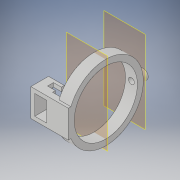
# Autodesk Inventor part: Dc_Ring
Saved by Autodesk Inventor 2019 (Build 230136000, 136)
## iProperties
Created: 2019-10-14
Part Number: Dc_Ring
Material: Generic
Document SubType Name: Modeling
Designer: James
Density: 1 g/cm^3
Appearance: Default
Author: James
Autodesk Inventor part; units mm, degrees
ref_plane "YZ Plane" through (0, 0, 0) normal (1, 0, 0) x (0, 1, 0)
ref_plane "XZ Plane" through (0, 0, 0) normal (0, 1, 0) x (-1, 0, 0)
sketch "Sketch1" plane through (0, 0, 0) normal (1, 0, 0) x (0, 1, 0)
  circle A0 centre (0, 0) radius 16
  circle A1 centre (0, 0) radius 19
  point P0 (19, 0)
  point P1 (0, -19)
  dimension "d0" = 32
  dimension "d1" = 3
  constraints: 2 centre point, 2 coincident, 2 point on circle
  measures "d0" diameter of A0
  measures "d1" radial gap between concentric circles of A1 A0
extrude "Extrusion1" add sketch "Sketch1" along normal blind 6
ref_plane "Work Plane2" through (0, 0, 19) normal (0, 0, 1) x (1, 0, 0)
sketch "Sketch4" plane through (0, 0, 19) normal (0, 0, 1) x (1, 0, 0)
  line L0 (6, 16) -> (6, -16) projected
  line L1 (6, 7) -> (-13, 7)
  line L2 (-13, 7) -> (-13, -7)
  line L3 (-13, -7) -> (6, -7)
  line L4 (6, -7) -> (6, 7)
  line L5 (-11, 5) -> (-5, 5)
  line L6 (-5, 5) -> (-5, -5)
  line L7 (-5, -5) -> (-11, -5)
  line L8 (-11, -5) -> (-11, 5)
  point P0 (0, 0)
  point P1 (-13, 0)
  point P2 (-5, 0)
  dimension "d11" = 14
  dimension "d12" = 19
  dimension "d13" = 6
  dimension "d14" = 10
  dimension "d15" = 2
  constraints: 16 end point, 4 parallel, 2 horizontal, 2 horizontal alignment, 2 midpoint, 2 perpendicular, 1 point on line
  measures "d11" distance of L1.end L2.end
  measures "d12" distance of L1.start L1.end
  measures "d13" distance of L5.start L5.end
  measures "d14" distance of L7.end L5.start
  measures "d15" distance between parallel lines of L2 L8
extrude "Extrusion4" add sketch "Sketch4" against normal blind 3
sketch "Sketch5" plane through (0, 0, 16) normal (0, 0, -1) x (-1, 0, 0)
  line L0 (13, 7) -> (13, -7) projected
  line L1 (13, -7) -> (-6, -7) projected
  line L2 (13, 7) -> (5, 7)
  line L3 (5, 7) -> (5, -7)
  line L4 (5, -7) -> (13, -7)
  line L5 (13, -7) -> (13, 7)
  line L6 (5, 5) -> (11, 5) projected
  line L7 (11, 5) -> (11, -5) projected
  line L8 (11, -5) -> (5, -5) projected
  point P0 (0, 0)
  constraints: 8 end point, 2 parallel, 2 point on line, 1 horizontal, 1 perpendicular
extrude "Extrusion5" add sketch "Sketch5" along normal blind 6 contours L0 L1 L3 L8 L7 L6 L2
sketch "Sketch6" plane through (-13, 7, 19) normal (0, 1, 0) x (1, 0, 0)
  line L0 (8, 3) -> (8, 9) projected
  line L1 (8, 7.5) -> (4, 7.5)
  line L2 (4, 7.5) -> (4, 4.5)
  line L3 (4, 4.5) -> (8, 4.5)
  line L4 (8, 4.5) -> (8, 7.5)
  line L5 (2, 0) -> (2, 9) projected
  line L6 (0, 9) -> (8, 9) projected
  point P0 (13, 19)
  dimension "d20" = 2
  dimension "d21" = 3
  dimension "d22" = 1.5
  constraints: 8 end point, 2 parallel, 1 horizontal, 1 perpendicular, 1 point on line
  measures "d20" distance between parallel lines of L5 L2
  measures "d21" distance between parallel lines of L3 L1
  measures "d22" distance between parallel lines of L6 L1
extrude "Extrusion6" cut sketch "Sketch6" against normal blind 17.25
ref_plane "Work Plane4" through (0, 0, -19) normal (0, 0, 1) x (1, 0, 0)
sketch "Sketch7" plane through (0, 0, -19) normal (0, 0, 1) x (1, 0, 0)
  circle A0 centre (3, 0) radius 1.5
  circle A1 centre (3, 0) radius 2.5
  line L0 (0, 19) -> (0, -19) projected
  point P0 (0, 0)
  point P1 (0, 0)
  point P2 (0, 7)
  point P3 (0, -7)
  dimension "d25" = 3
  dimension "d26" = 5
  dimension "d27" = 3
  constraints: 2 centre point, 1 coincident, 1 horizontal alignment, 1 midpoint
  measures "d25" diameter of A0
  measures "d26" diameter of A1
  measures "d27" distance of point (0, 0) A0.centre
extrude "Extrusion7" add sketch "Sketch7" along normal mid plane 6
sketch "Sketch8" plane through (3, 0, -22) normal (0, 0, -1) x (-1, 0, 0)
  circle A0 centre (0, 0) radius 1.5 projected
  point P0 (3, 0)
extrude "Extrusion8" cut sketch "Sketch8" against normal blind 10.75
body "Solid1"
